Autodesk Fusion 360 part; units mm, degrees
note: some values were not read from the file. Set by a fixed rule: which face or edge a step refers to.
(part 2 of 2)
extrude "Extrude38" add sketch "Sketch20" along normal blind 2.5 contours L1 L6 S3 S5 | L1 L4 L5 S2 S3 L13 L14 L15 S4 L26 L27 L28 S5 | L6 S3 L22 L25 S5 L29 | L1 L8 S2 S4 | L8 S2 L21 L25 S4 L30 bodies 6
combine "Combine5" operation cut target body 1 tool bodies 6 keep tools
sketch "Sketch21" plane through (112.7, 0, 0) normal (1, 0, 0) x (0, 1, 0)
  line L0 (8.1693, -6.4) -> (8.1693, 0)
  line L1 (8.1693, 0) -> (64.35, 0)
  line L2 (64.35, 0) -> (64.35, 6.9)
  line L3 (64.35, 6.9) -> (64.35, 12.2)
  line L4 (64.35, 12.2) -> (0, 12.2)
  line L5 (0, 12.2) -> (0, 0)
  arc A0 (0, 0) -> (6.4, -6.4) centre (6.4, 0) ccw
  line L6 (6.4, -6.4) -> (8.1693, -6.4)
extrude "Extrude39" cut sketch "Sketch7" against normal blind 8.619 contours A0 L3 L4 L6 | A0 bodies 6
extrude "Extrude40" cut sketch "Sketch8" along normal blind 3.572 and the other way blind 5.796 contours A1 L17 L24 L25 L30 | A0 L8 A1 L16 L25 L26 L30 bodies 6
chamfer "Chamfer4" distance 1.4 angle 45 2 edges at (107.005, 116.4968, 8.25) (107.005, 116.4968, 4.5111) tangent chain off on bodies 1
chamfer "Chamfer5" distance 0.763 angle 45 7 edges at (107.0073, 100.9269, 8.7307) (107.005, 103.3433, 5.278) (107.0073, 100.9268, 1.8252) (107.0557, 96.993, 1.603) (107.2633, 91.1985, 3.3357) (107.206, 92.3759, 8.3977) (107.0557, 96.993, 8.953) tangent chain off on bodies 1
fillet "Fillet2" radius 0.937 4 edges at (105.185, 101.5433, 6.943) (105.185, 92.4433, 6.943) (104.615, 101.5433, 3.613) (104.615, 92.4433, 3.613) on bodies 1
chamfer "Chamfer6" distance 0.754 angle 45 2 edges at (103.865, 92.1933, 6.943) (103.865, 101.7933, 6.943) tangent chain off on bodies 1
chamfer "Chamfer7" distance 1.611 angle 45 2 edges at (0, 44.7383, 8.528) (0, 44.7383, 5.9361) tangent chain off on bodies 1
extrude "Extrude41" add sketch "Sketch16" against normal blind 0.6 separate body contours S2 S3 S4 L18 S5 S6 S7 S8 S9 S10 S11 S12 S13 S14 S15 S16 S17 S18 S19 S20 L19 S21 S22 S23 S24 S25 S26 S27 S28 S29 S30 S31 S32 S33 | S34 S35 S36 S37 S38 S39 S40 S41 S42 S43 S44 S45 | S58 S59 S60 L20 L21 L22 S61 S62 S63 S64 L23 S65 S66 | S67 S68 S69 S70 S71 S72 S73 S74 | S75 S76 S77 L24 S78 S79 S80 S81 S82 S83 L25 S84 S85 S86 | L27 S96 L28 L29 L31 | L26 S90 L27 S96 L29 L31 | L26 S90 L29 L30 L31 | L32 L40 L41 L43 | L32 L38 L39 L41 L43 | L32 L33 L34 | L32 L34 L35 L36 L37 L38 L41 | L38 L41 L42 L43 makes body 7 at (19.56, 60.7094, 12.2) makes body 8 at (26.269, 60.3587, 12.2) makes body 9 at (17.9961, 59.989, 12.2) makes body 10 at (22.9273, 59.2688, 12.2) makes body 11 at (29.6436, 61.0915, 12.2) makes body 12 at (14.2114, 60.1901, 12.2)
hidden bodies 2 6
equation "d12 = outer_spacing"
equation "outer_spacing = 2 mm"
equation "d14 = outer_spacing"
equation "d17 = outer_spacing"
equation "d21 = outer_spacing"
equation "d22 = outer_spacing"
equation "topmost_wall_thickness = 0,75 mm"
equation "top_support_wall_tickness = 5,3 mm"
equation "bottom_wall_thickness = 3 mm"
equation "d27 = topmost_wall_thickness"
equation "d28 = top_support_wall_tickness"
equation "d29 = top_support_wall_tickness"
equation "d55 = outer_spacing"
equation "d229 = outer_spacing"
equation "d230 = -outer_spacing"
equation "d235 = -outer_spacing / 2"
